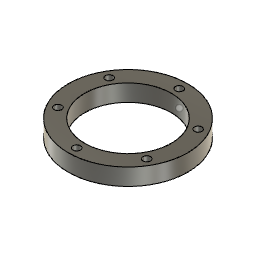
Lochsirenenring_v3 (Autodesk Fusion 360 design; units mm, degrees)
Autodesk Fusion 360 part; units mm, degrees
sketch "Sketch17" plane through (0, 0, 0) normal (0, 0, 1) x (1, 0, 0)
  circle A0 centre (0, 0) radius 25.75
  circle A1 centre (0, 0) radius 35.5
  dimension "d61" = 51.5
  dimension "d62" = 71
  constraint coincident A0.centre A1.centre
  constraint concentric A0 A1
  measures "d61" diameter of A0
  measures "d62" diameter of A1
extrude "Extrude10" add sketch "Sketch17" along normal blind 10
sketch "Sketch18" plane through (0, 0, 0) normal (0, 0, 1) x (1, 0, 0)
  point P0 (0, 30.5)
sketch "Sketch19" plane through (0, 0, 0) normal (0, 0, 1) x (1, 0, 0)
  circle A0 centre (0, 30.5) radius 2.25
  dimension "d65" = 4.5
  measures "d65" diameter of A0
extrude "Extrude11" cut sketch "Sketch19" along normal blind 10
pattern_circular "C-Pattern7" count 6 over 360 about axis through (0, 0, 0) along (0, 0, 1) of "Extrude11"
